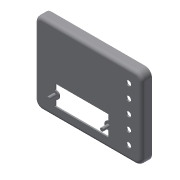
# Autodesk Inventor part: 4600-2358
Saved by Autodesk Inventor 2022 (Build 260148000, 148)
## iProperties
Shininess: 64.0
Length Units: 11269
Angle Units: 11279
Time Units: 11290
Mass Units: 11283
Length Display Precision: 3
Angle Display Precision: 2
Created: 2002-04-17
Part Number: 4600-2358
Document SubType Name: Modeling
Designer: Administrator
Density: 1 g/cm^3
Material: Generic
Appearance: Default
Density: 0.0
Volumn: 0.0
Area: 0.0
PropertySet Name: Model Information
Control State: 0
Master: False
Checked Out: False
Author: Administrator
Autodesk Inventor part; units mm, degrees
ref_plane "YZ Plane" through (0, 0, 0) normal (1, 0, 0) x (0, 1, 0)
ref_plane "XZ Plane" through (0, 0, 0) normal (0, 1, 0) x (-1, 0, 0)
ref_plane "XY Plane" through (0, 0, 0) normal (0, 0, 1) x (1, 0, 0)
sketch "Sketch1" plane through (0, 0, 0) normal (0, 0, 1) x (1, 0, 0)
  line L0 (-16.0584, 31.8961) -> (85.5416, 31.8961)
  line L1 (85.5416, 31.8961) -> (85.5416, -44.4039)
  line L2 (85.5416, -44.4039) -> (-16.0584, -44.4039)
  line L3 (-16.0584, -44.4039) -> (-16.0584, 31.8961)
  dimension "d0" = 101.6
  dimension "d1" = 76.3
  constraints: 8 end point, 2 parallel, 1 horizontal, 1 perpendicular
  measures "d0" distance of L1.end L2.end
  measures "d1" distance of L2.end L0.start
extrude "Extrusion1" add sketch "Sketch1" along normal blind 9.525
fillet "Fillet1" radius 6.35 4 edges at (85.5416, 31.8961, 4.7625) (85.5416, -44.4039, 4.7625) (-16.0584, -44.4039, 4.7625) (-16.0584, 31.8961, 4.7625)
fillet "Fillet2" radius 3.175 8 edges at (34.7416, 31.8961, 9.525) (83.6817, 30.0362, 9.525) (85.5416, -6.2539, 9.525) (83.6817, -42.544, 9.525) (34.7416, -44.4039, 9.525) (-14.1985, -42.544, 9.525) (-16.0584, -6.2539, 9.525) (-14.1985, 30.0362, 9.525)
shell "Shell1" thickness 1.27 removed faces 1 at (49.5583, -18.9706, 0)
sketch "Sketch2" plane through (0, 0, 9.525) normal (0, 0, 1) x (1, 0, 0)
  circle A0 centre (2.9916, -25.3539) radius 1.5875
  line L0 (-16.0584, 25.5461) -> (-16.0584, -38.0539) projected
  line L1 (-9.7084, -44.4039) -> (79.1916, -44.4039) projected
  dimension "d7" = 3.175
  dimension "d8" = 19.05
  dimension "d9" = 19.05
  constraints: 1 centre point
  measures "d7" diameter of A0
  measures "d8" distance from line of L0 A0.centre
  measures "d9" distance from line of L1 A0.centre
extrude "Extrusion2" add sketch "Sketch2" along normal blind 6.35
pattern_linear "Rectangular Pattern1" count 2 spacing 50.8 along (1, 0, 0) of "Extrusion2"
sketch "Sketch3" plane through (0, 0, 9.525) normal (0, 0, 1) x (1, 0, 0)
  line L0 (82.3666, 25.5461) -> (82.3666, -38.0539) projected
  line L1 (2.9916, -15.8289) -> (2.9916, -21.5439)
  arc A0 (2.9916, -29.1639) -> (2.9916, -21.5439) centre (2.9916, -25.3539) ccw
  line L2 (2.9916, -29.1639) -> (2.9916, -34.8789)
  line L3 (2.9916, -34.8789) -> (53.7916, -34.8789)
  line L4 (53.7916, -34.8789) -> (53.7916, -29.1639)
  arc A1 (53.7916, -21.5439) -> (53.7916, -29.1639) centre (53.7916, -25.3539) ccw
  line L5 (53.7916, -21.5439) -> (53.7916, -15.8289)
  line L6 (53.7916, -15.8289) -> (2.9916, -15.8289)
  circle A2 centre (2.9916, -25.3539) radius 1.5875 projected
  circle A3 centre (53.7916, -25.3539) radius 1.5875 projected
  dimension "d15" = 19.05
  dimension "d17" = 3.81
  constraints: 12 end point, 4 collinear, 4 parallel, 4 point on circle, 2 centre point, 2 concentric, 2 point on line, 1 equal radius, 1 perpendicular
  measures "d15" distance of L1.start L2.end
  measures "d17" radius of A0
extrude "Extrusion3" cut sketch "Sketch3" against normal blind 6.35 contours L6 L5 A1 L4 L3 L2 A0 L1
sketch "Sketch4" plane through (0, 0, 9.525) normal (0, 0, 1) x (1, 0, 0)
  line L0 (85.5416, -38.0539) -> (85.5416, 25.5461) projected
  line L1 (-9.7084, -44.4039) -> (79.1916, -44.4039) projected
  point P0 (72.8416, -31.7039)
  dimension "d20" = 12.7
  dimension "d21" = 12.7
  measures "d20" distance from line of L0 point (72.842, -31.704)
  measures "d21" distance from line of point (72.842, -31.704) L1
hole "Hole1" at (72.8416, -31.7039, 9.525) direction (0, 0, -1) diameter 4.7752 end through all
pattern_linear "Rectangular Pattern2" count 5 spacing 12.7 along (0, 1, 0) of "Hole1"
body "Solid1"
